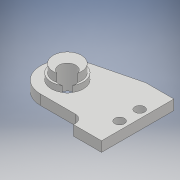
# Autodesk Inventor part: MCP mount M F5
Saved by Autodesk Inventor 2017 (Build 210142000, 142)
## iProperties
Created: 2018-07-27
Part Number: MCP mount M F5
Material: Generic
Document SubType Name: Modeling
Designer: jakub.tomczynski
Density: 1 g/cm^3
Appearance: Default
Author: jakub.tomczynski
## iProperties of the stored document MCP mount M F5_3DPrint.ipt
Created: 2018-09-03
Part Number: MCP mount M F5_3DPrint
Material: Generic
Document SubType Name: Modeling
Designer: jakub.tomczynski
Density: 1 g/cm^3
Appearance: Default
Author: jakub.tomczynski
Autodesk Inventor part; units mm, degrees
ref_plane "YZ Plane" through (0, 0, 0) normal (1, 0, 0) x (0, 1, 0)
ref_plane "XZ Plane" through (0, 0, 0) normal (0, 1, 0) x (-1, 0, 0)
ref_plane "XY Plane" through (0, 0, 0) normal (0, 0, 1) x (1, 0, 0)
sketch "MCP joint" plane through (0, 0, 0) normal (0, 0, 1) x (1, 0, 0)
  point P0 (0, 0)
  point P1 (0, 0)
  constraints: 1 coincident
sketch "Sketch2" plane through (0, 0, 0) normal (0, 0, 1) x (1, 0, 0)
  line L0 (9, -7.5) -> (16, -7.5)
  line L1 (16, -7.5) -> (16, 10.5)
  line L2 (16, 10.5) -> (9, 10.5)
  circle A0 centre (0, 0) radius 8
  line L3 (9, 10.5) -> (-1.9428, 7.7605)
  line L4 (9, -7.5) -> (0.4552, -7.987)
  point P0 (16, 1.5)
  point P1 (3.5, 1.5)
  point P2 (16, 1.5)
  dimension "d0" = 18
  dimension "d3" = 16
  dimension "d94" = 1.5
  dimension "d95" = 16
  dimension "d96" = 9
  dimension "d97" = 9
  constraints: 10 end point, 2 coincident, 2 point on circle, 2 tangent, 1 centre point, 1 horizontal, 1 midpoint, 1 parallel, 1 perpendicular
  measures "d0" distance between parallel lines of L0 L2
  measures "d3" distance from line of L1 point (0, 0)
  measures "d94" vertical distance of point (0, 0) point (16, 1.5)
  measures "d95" diameter of A0
  measures "d96" horizontal distance of L2.end point (0, 0)
  measures "d97" horizontal distance of L0.start point (0, 0)
extrude "base" add sketch "Sketch2" along normal blind 2.5
sketch "Sketch3" plane through (0, 0, 2.5) normal (0, 0, 1) x (1, 0, 0)
  point P0 (0, 0)
  point P1 (0, 0)
hole "bearing pocket" at (0, 0, 2.5) direction (0, 0, -1) diameter 4 end through all
sketch "Sketch13" plane through (0, 0, 0) normal (0, 0, -1) x (-1, 0, 0)
  line L0 (-9, -7.5) -> (-9, -5)
  arc A0 (-0.4552, -7.987) -> (1.9428, 7.7605) centre (0, 0) ccw projected
  line L1 (-9, -5) -> (6.245, -5)
  line L2 (-0.4552, -7.987) -> (-9, -7.5) projected
  dimension "d76" = 2.5
  constraints: 4 end point, 1 horizontal, 1 point on circle, 1 vertical
  measures "d76" distance of L0.start L0.end
extrude "bottom cutout" cut sketch "Sketch13" against normal through all
fillet "Fillet2" radius 2 1 edges at (9, -5, 1.25)
fillet "Fillet4" radius 6 1 edges at (-6.245, -5, 1.25)
sketch "Sketch7" plane through (0, 0, 0) normal (0, 0, -1) x (-1, 0, 0)
  line L0 (3, 2.5) -> (-4.5, 2.5) construction
  line L1 (-4.5, 2.5) -> (-4.5, -2.5) construction
  line L2 (-4.5, -2.5) -> (3, -2.5) construction
  line L3 (3, -2.5) -> (3, 2.5) construction
  line L4 (3, 2.5) -> (-4.5, -2.5) construction
  line L5 (-4.5, 2.5) -> (3, -2.5) construction
  point P0 (0, 0)
  point P1 (-0.75, 0)
  point P2 (0, 0)
  point P3 (-0.75, 0)
  dimension "d34" = 3
  dimension "d35" = 4.5
  dimension "d36" = 5
  constraints: 12 end point, 3 midpoint, 2 parallel, 1 horizontal, 1 horizontal alignment, 1 perpendicular
  measures "d34" distance from line of point (0, 0) L3
  measures "d35" distance from line of L1 point (0, 0)
  measures "d36" distance between parallel lines of L2 L0
hole "potentiometer pins" at (-3, 2.5, 0) at (-3, -2.5, 0) at (4.5, -2.5, 0) at (4.5, 2.5, 0) direction (0, 0, 1) diameter 1 depth 1.5
sketch "Sketch8" plane through (0, 0, 2.5) normal (0, 0, 1) x (1, 0, 0)
  line L0 (8.1428, 0) -> (0, 0) construction
  line L1 (0, 0) -> (-8.8782, 8.8782) construction
  circle A0 centre (-1.4142, 1.4142) radius 3.5
  dimension "d45" = 2
  dimension "d46" = 7
  dimension "d59" = 45
  constraints: 4 end point, 1 centre point, 1 coincident, 1 horizontal, 1 point on line
  measures "d45" distance of A0.centre point (0, 0)
  measures "d46" diameter of A0
  measures "d59" angle of L0 L1
extrude "bearing" add sketch "Sketch8" along normal blind 3.5
sketch "Sketch10" plane through (0, 0, 2.5) normal (0, 0, 1) x (1, 0, 0)
  circle A0 centre (-1.4142, 1.4142) radius 3.5 projected
  circle A1 centre (-1.4142, 1.4142) radius 4
  point P0 (0, 0)
  point P1 (1.0607, -1.0607)
  dimension "d56" = 8
  constraints: 1 centre point, 1 coincident, 1 other
  measures "d56" diameter of A1
extrude "bearing spacer" add sketch "Sketch10" along normal blind 1.5
sketch "Sketch11" plane through (-1.4142, 1.4142, 6) normal (0, 0, 1) x (1, 0, 0)
  point P0 (1.4142, -1.4142)
  point P1 (1.4142, -1.4142)
hole "Hole4" at (0, 0, 6) direction (0, 0, -1) diameter 4.2 end through all
sketch "Sketch12" plane through (0, 0, 2.5) normal (0, 0, 1) x (1, 0, 0)
  point P0 (0, 0)
  point P1 (14, 4)
  point P2 (14, -1)
  point P3 (0, 0)
  dimension "d88" = 14
  dimension "d89" = 14
  dimension "d90" = 4
  dimension "d91" = 1
  measures "d88" horizontal distance of point (14, 4) point (0, 0)
  measures "d89" horizontal distance of point (14, -1) point (0, 0)
  measures "d90" vertical distance of point (14, 4) point (0, 0)
  measures "d91" vertical distance of point (14, -1) point (0, 0)
hole "mounting" at (14, 4, 2.5) at (14, -1, 2.5) direction (0, 0, -1) diameter 2.4 end through all
equation "\"d45\" = MCP_spring_arm"
equation "\"MCP_spring_arm\" = F5_MCP_spring_arm"
equation "\"F5_MCP_spring_arm\" = 2"
body "Solid1"
